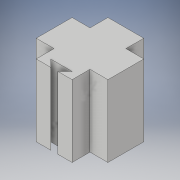
# Autodesk Inventor part: test3
Saved by Autodesk Inventor 2018.2 (Build 222227000, 227)
## iProperties
Created: 2018-03-29
Part Number: test3
Material: Generic
Document SubType Name: Modeling
Designer: martin
Density: 1 g/cm^3
Appearance: Default
Author: martin
Autodesk Inventor part; units mm, degrees
ref_plane "YZ Plane" through (0, 0, 0) normal (1, 0, 0) x (0, 1, 0)
ref_plane "XZ Plane" through (0, 0, 0) normal (0, 1, 0) x (-1, 0, 0)
ref_plane "XY Plane" through (0, 0, 0) normal (0, 0, 1) x (1, 0, 0)
sketch "Sketch1" plane through (0, 0, 0) normal (0, 1, 0) x (-1, 0, 0)
  line L0 (-25.4, -12.7) -> (25.4, -12.7)
  line L1 (25.4, -12.7) -> (25.4, 12.7)
  line L2 (25.4, 12.7) -> (-25.4, 12.7)
  line L3 (-25.4, 12.7) -> (-25.4, -12.7)
  line L4 (-25.4, -12.7) -> (25.4, 12.7) construction
  line L5 (25.4, -12.7) -> (-25.4, 12.7) construction
  point P0 (0, 0)
  dimension "d0" = 25.4
  dimension "d1" = 50.8
  constraints: 12 end point, 2 midpoint, 2 parallel, 1 horizontal, 1 perpendicular
  measures "d0" distance of L0.end L1.end
  measures "d1" distance of L0.start L0.end
extrude "Extrusion1" add sketch "Sketch1" along normal mid plane 50.8
sketch "Sketch2" plane through (-25.4, 25.4, 12.7) normal (0, 0, 1) x (1, 0, 0)
  line L0 (50.8, 0) -> (0, 0) projected
  line L1 (38.1, -50.8) -> (12.7, -50.8)
  line L2 (12.7, -50.8) -> (12.7, 0)
  line L3 (12.7, 0) -> (38.1, 0)
  line L4 (38.1, 0) -> (38.1, -50.8)
  line L5 (38.1, -50.8) -> (12.7, 0) construction
  line L6 (12.7, -50.8) -> (38.1, 0) construction
  point P0 (25.4, -25.4)
  dimension "d4" = 50.8
  dimension "d5" = 25.4
  constraints: 12 end point, 2 midpoint, 2 parallel, 1 horizontal, 1 perpendicular, 1 point on line
  measures "d4" distance between parallel lines of L1 L3
  measures "d5" distance between parallel lines of L4 L2
extrude "Extrusion2" add sketch "Sketch2" along normal blind 12.7 and the other way blind 38.1
sketch "Sketch3" plane through (0, -25.4, 0) normal (0, -1, 0) x (1, 0, 0)
  line L0 (12.7, 25.4) -> (-12.7, 25.4) projected
  line L1 (0, 25.4) -> (-2.4016, 25.4)
  line L2 (-7.4816, 20.32) -> (7.7584, 20.32)
  line L3 (7.7584, 20.32) -> (2.6784, 25.4)
  line L4 (-2.4016, 25.4) -> (-7.4816, 20.32)
  point P0 (0, 0)
  dimension "d10" = 5.08
  dimension "d11" = 5.08
  dimension "d12" = 15.24
  dimension "d13" = 45
  dimension "d14" = 25.4
  dimension "d15" = 45
  constraints: 8 end point, 2 point on line, 1 midpoint
  measures "d10" distance from line of L0 L2.start
  measures "d11" distance from line of L0 L2.end
  measures "d12" distance of L2.start L2.end
  measures "d13" angle of L0 L3
  measures "d14" distance of L0.start L0.end
  measures "d15" angle of L0 L4
extrude "Extrusion3" cut sketch "Sketch3" against normal up to next
body "Solid1"
